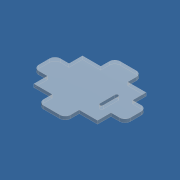
# Autodesk Inventor part: Front_stopper
Saved by Autodesk Inventor 2016 (Build 200138000, 138)
## iProperties
Created: 2016-04-04
Part Number: Front_stopper
Material: Polycarbonate, Clear
Document SubType Name: Modeling
Designer: admin
Density: 1.2 g/cm^3
Appearance: Polycarbonate - Clear
Author: admin
Autodesk Inventor part; units mm, degrees
ref_plane "YZ Plane" through (0, 0, 0) normal (1, 0, 0) x (0, 1, 0)
ref_plane "XZ Plane" through (0, 0, 0) normal (0, 1, 0) x (-1, 0, 0)
ref_plane "XY Plane" through (0, 0, 0) normal (0, 0, 1) x (1, 0, 0)
sketch "Sketch1" plane through (0, 0, 0) normal (0, 0, 1) x (1, 0, 0)
  line L0 (-12.5, 22.5) -> (-12.5, 30.5)
  line L1 (-7.5, 35.5) -> (7.5, 35.5)
  line L2 (12.5, 30.5) -> (12.5, 22.5)
  line L3 (-12.5, -22.5) -> (-12.5, -30.5)
  line L4 (-7.5, -35.5) -> (7.5, -35.5)
  line L5 (12.5, -30.5) -> (12.5, -22.5)
  line L6 (29.5, 10) -> (37.5, 10)
  line L7 (42.5, 5) -> (42.5, -5)
  line L8 (37.5, -10) -> (29.5, -10)
  line L9 (-29.5, 10) -> (-37.5, 10)
  line L10 (-42.5, 5) -> (-42.5, -5)
  line L11 (-37.5, -10) -> (-29.5, -10)
  arc A0 (-7.5, 35.5) -> (-12.5, 30.5) centre (-7.5, 30.5) ccw
  arc A1 (12.5, 30.5) -> (7.5, 35.5) centre (7.5, 30.5) ccw
  arc A2 (-37.5, 10) -> (-42.5, 5) centre (-37.5, 5) ccw
  arc A3 (-42.5, -5) -> (-37.5, -10) centre (-37.5, -5) ccw
  arc A4 (-12.5, -30.5) -> (-7.5, -35.5) centre (-7.5, -30.5) ccw
  arc A5 (7.5, -35.5) -> (12.5, -30.5) centre (7.5, -30.5) ccw
  arc A6 (37.5, -10) -> (42.5, -5) centre (37.5, -5) ccw
  arc A7 (42.5, 5) -> (37.5, 10) centre (37.5, 5) ccw
  line L12 (-29.5, 22.5) -> (-12.5, 22.5)
  line L13 (12.5, 22.5) -> (29.5, 22.5)
  line L14 (-29.5, -22.5) -> (-29.5, -10)
  line L15 (-29.5, 10) -> (-29.5, 22.5)
  line L16 (29.5, -22.5) -> (12.5, -22.5)
  line L17 (-12.5, -22.5) -> (-29.5, -22.5)
  line L18 (29.5, 22.5) -> (29.5, 10)
  line L19 (29.5, -10) -> (29.5, -22.5)
  point P0 (0, 0)
  point P1 (29.5, 0)
  point P2 (0, 22.5)
  point P3 (-12.5, -35.5)
  point P4 (12.5, -35.5)
  point P5 (-42.5, 10)
  point P6 (-42.5, -10)
  point P7 (-42.5, 0)
  point P8 (0, 35.5)
  dimension "d0" = 45
  dimension "d1" = 59
  dimension "d2" = 5
  dimension "d3" = 13
  dimension "d4" = 25
  dimension "d5" = 20
  constraints: 40 end point, 16 point on circle, 16 point on line, 16 tangent, 12 perpendicular, 8 centre point, 8 parallel, 7 equal radius, 5 equal length, 4 collinear, 3 horizontal, 2 horizontal alignment, 2 midpoint, 2 vertical alignment, 1 vertical
  measures "d0" distance of L14.start L12.start
  measures "d1" distance of L16.start L14.start
  measures "d2" radius of A0
  measures "d3" distance between parallel lines of L13 L1
  measures "d4" distance between parallel lines of L2 L0
  measures "d5" distance between parallel lines of L8 L6
extrude "Extrusion1" add sketch "Sketch1" along normal blind 3
sketch "Sketch2" plane through (0, 0, 3) normal (0, 0, 1) x (1, 0, 0)
  line L0 (19.8902, 6.2991) -> (19.8902, -7.8023)
  line L1 (16.8902, -7.8023) -> (16.8902, 6.2991)
  arc A0 (19.8902, 6.2991) -> (16.8902, 6.2991) centre (18.3902, 6.2991) ccw
  arc A1 (16.8902, -7.8023) -> (19.8902, -7.8023) centre (18.3902, -7.8023) ccw
  point P0 (0, 0)
  dimension "d8" = 3
  constraints: 4 end point, 4 point on circle, 4 tangent, 2 centre point, 1 parallel
  measures "d8" distance between parallel lines of L1 L0
extrude "Extrusion2" cut sketch "Sketch2" against normal blind 10
body "Solid1"
